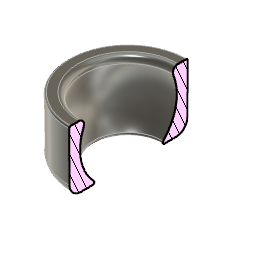
Mazda MX5 NB Shift Cup R1 (Autodesk Fusion 360 design; units mm, degrees)
Autodesk Fusion 360 part; units mm, degrees
sketch "Cup" plane through (0, 0, 0) normal (0, 0, 1) x (1, 0, 0)
  circle A0 centre (0, 0) radius 10.5
  circle A1 centre (0, 0) radius 5.75
  circle A2 centre (0, 0) radius 7.75
  dimension "d6" = 21
  dimension "d9" = 11.5
  dimension "d10" = 15.5
  dimension "d11" = 5.5
  constraint coincident A0.centre A1.centre
  constraint concentric A0 A1
  measures "d6" diameter of A0
  measures "d9" diameter of A1
  measures "d10" diameter of A2
  measures "d11" distance of A0.centre A1.centre
extrude "Extrude Cup" add sketch "Cup" against normal blind 11 draft -0.5 from surface at 11 contours A0 | A1 | A2
sphere "Negative Extrude Ball" cut diameter 17.1 placed x (1, 0, 0) y (0, 0, -1) z (0, 1, 0) at (0, 0, 6.5)
extrude "Negative Extrude Lower Lip" cut sketch "Cup" along normal blind 1.5 contours A1
extrude "Negative Extrude Upper Lip" cut sketch "Cup" along normal blind 6 from surface at 5.5 contours A2
fillet "Fillet3" radius 2 1 edges at (-9.6999, -3.7622, 0)
fillet "Fillet3" radius 0.9 1 faces at (7.7115, 0.7717, 10.4074)
fillet "Fillet3" radius 0.3 1 edges at (-9.7894, -3.797, 11) 1 faces at (5.7214, 0.5725, 0.1149)
named bodies: "Cup"
